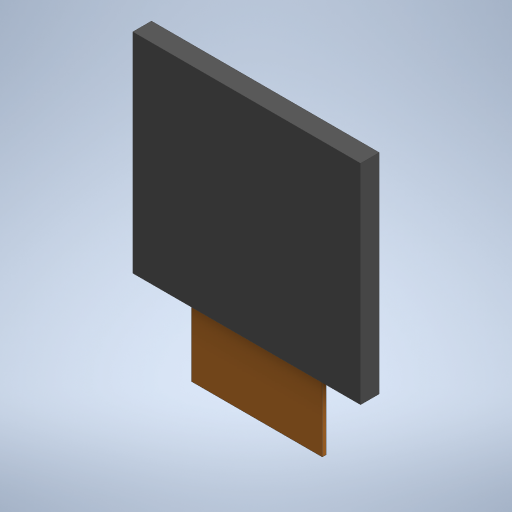
# Autodesk Inventor part: 0_42_oled
Saved by Autodesk Inventor 2023 (Build 270158000, 158)
## iProperties
Created: 2024-03-19
Part Number: 0_42_oled
Material: Generic
Document SubType Name: Modeling
Designer: noname
Density: 1 g/cm^3
Appearance: Default
Author: noname
Autodesk Inventor part; units mm, degrees
ref_plane "YZ Plane" through (0, 0, 0) normal (1, 0, 0) x (0, 1, 0)
ref_plane "XZ Plane" through (0, 0, 0) normal (0, 1, 0) x (-1, 0, 0)
sketch "Sketch2" plane through (0, 0, 0) normal (0, 0, 1) x (1, 0, 0)
  line L0 (-6.1, 0) -> (6.1, 0)
  line L1 (6.1, 0) -> (6.1, 11.2)
  line L2 (6.1, 11.2) -> (-6.1, 11.2)
  line L3 (-6.1, 11.2) -> (-6.1, 0)
  point P0 (0, 0)
  point P1 (0, 0)
  dimension "d0" = 12.2
  dimension "d1" = 11.2
  constraints: 8 end point, 2 parallel, 1 coincident, 1 horizontal, 1 midpoint, 1 perpendicular
  measures "d0" distance between parallel lines of L1 L3
  measures "d1" distance between parallel lines of L0 L2
extrude "Extrusion1" add sketch "Sketch2" along normal blind 1
ref_plane "Work Plane1" through (0, 0, 0.25) normal (0, 0, -1) x (-1, 0, 0)
sketch "Sketch3" plane through (0, 0, 0.25) normal (0, 0, -1) x (-1, 0, 0)
  line L0 (-3.5, 0) -> (3.5, 0)
  line L1 (3.5, 0) -> (3.5, -4)
  line L2 (3.5, -4) -> (-3.5, -4)
  line L3 (-3.5, -4) -> (-3.5, 0)
  line L4 (6.1, 0) -> (-6.1, 0) projected
  point P0 (0, 0)
  point P1 (0, 0)
  dimension "d5" = 4
  dimension "d6" = 7
  constraints: 8 end point, 2 midpoint, 2 parallel, 1 horizontal, 1 perpendicular
  measures "d5" distance between parallel lines of L0 L2
  measures "d6" distance between parallel lines of L1 L3
extrude "Extrusion2" add sketch "Sketch3" against normal blind 0.2
body "Solid1"
